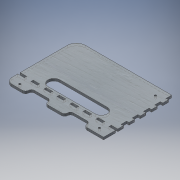
# Autodesk Inventor part: LatoPy
Saved by Autodesk Inventor 2018.3 (Build 223284000, 284)
## iProperties
Created: 2019-03-05
Part Number: LatoPy
Material: Generico
Document SubType Name: Modeling
Designer: AlfyPc
Density: 1 g/cm^3
Appearance: Legno - Verniciato - Bianco
Author: AlfyPc
Autodesk Inventor part; units mm, degrees
ref_plane "YZ Plane" through (0, 0, 0) normal (1, 0, 0) x (0, 1, 0)
ref_plane "XZ Plane" through (0, 0, 0) normal (0, 1, 0) x (-1, 0, 0)
ref_plane "XY Plane" through (0, 0, 0) normal (0, 0, 1) x (1, 0, 0)
sketch "Schizzo1" plane through (0, 0, 0) normal (0, 0, 1) x (1, 0, 0)
  line L0 (4, 17) -> (0, 17) construction
  line L1 (0, 17) -> (0, 95) construction
  line L2 (0, 95) -> (4, 95) construction
  line L3 (4, 95) -> (4, 17) construction
  line L4 (4, -4) -> (4, -24) construction
  line L5 (4, -24) -> (0, -24) construction
  line L6 (0, -24) -> (0, -4) construction
  line L7 (0, 0) -> (0, 11) construction
  line L8 (0, 11) -> (4, 11) construction
  line L9 (4, 11) -> (4, 0) construction
  line L10 (-161, -24) -> (-161, 95)
  line L11 (-161, 95) -> (4, 95)
  line L12 (4, 95) -> (4, -24)
  line L13 (-133, -24) -> (-161, -24)
  arc A0 (-133, -24) -> (-128, -19) centre (-133, -19) ccw
  arc A1 (-123, -14) -> (-128, -19) centre (-123, -19) ccw
  line L14 (-100, -14) -> (-123, -14)
  arc A2 (-95, -19) -> (-100, -14) centre (-100, -19) ccw
  arc A3 (-95, -19) -> (-90, -24) centre (-90, -19) ccw
  line L15 (-67, -24) -> (-90, -24)
  arc A4 (-67, -24) -> (-62, -19) centre (-67, -19) ccw
  arc A5 (-57, -14) -> (-62, -19) centre (-57, -19) ccw
  line L16 (-34, -14) -> (-57, -14)
  arc A6 (-29, -19) -> (-34, -14) centre (-34, -19) ccw
  arc A7 (-29, -19) -> (-24, -24) centre (-24, -19) ccw
  line L17 (4, -24) -> (-24, -24)
  line L18 (-117, 13) -> (-37, 13) construction
  line L19 (-117, 3) -> (-37, 3)
  line L20 (-37, 23) -> (-117, 23)
  arc A8 (-117, 23) -> (-117, 3) centre (-117, 13) ccw
  arc A9 (-37, 3) -> (-37, 23) centre (-37, 13) ccw
  line L21 (-161, -4) -> (-150, -4) projected
  line L22 (-150, 0) -> (-150, -4) projected
  line L23 (-139, -4) -> (-128, -4) projected
  line L24 (-128, 0) -> (-128, -4) projected
  line L25 (-139, 0) -> (-128, 0) projected
  line L26 (-139, 0) -> (-139, -4) projected
  line L27 (-117, -4) -> (-106, -4) projected
  line L28 (-106, 0) -> (-106, -4) projected
  line L29 (-117, 0) -> (-106, 0) projected
  line L30 (-117, 0) -> (-117, -4) projected
  line L31 (-95, -4) -> (-84, -4) projected
  line L32 (-84, 0) -> (-84, -4) projected
  line L33 (-95, 0) -> (-84, 0) projected
  line L34 (-95, 0) -> (-95, -4) projected
  line L35 (-73, -4) -> (-62, -4) projected
  line L36 (-62, 0) -> (-62, -4) projected
  line L37 (-73, 0) -> (-62, 0) projected
  line L38 (-73, 0) -> (-73, -4) projected
  line L39 (-51, -4) -> (-40, -4) projected
  line L40 (-40, 0) -> (-40, -4) projected
  line L41 (-51, 0) -> (-40, 0) projected
  line L42 (-51, 0) -> (-51, -4) projected
  line L43 (-29, -4) -> (-18, -4) projected
  line L44 (-18, 0) -> (-18, -4) projected
  line L45 (-29, 0) -> (-18, 0) projected
  line L46 (-29, 0) -> (-29, -4) projected
  line L47 (-7, -4) -> (4, -4) projected
  line L48 (4, 0) -> (4, -4) projected
  line L49 (-7, 0) -> (4, 0) projected
  line L50 (-7, 0) -> (-7, -4) projected
  line L51 (-161, 0) -> (-150, 0) projected
  line L52 (-161, 0) -> (-161, -4) projected
  point P0 (-77, 13)
  dimension "d0" = 80
  constraints: 44 end point, 20 point on circle, 10 centre point, 6 vertical, 4 horizontal, 4 tangent, 2 parallel, 1 midpoint, 10 other
  measures "d0" distance of L18.start L18.end
extrude "Estrusione1" add sketch "Schizzo1" along normal blind 4 contours L10 L21 L22 L51 L11 L12 L49 L50 L47 L17 A7 A6 L16 A5 A4 L15 A3 A2 L14 A1 A0 L13
sketch "Schizzo2" plane through (0, 0, 4) normal (0, 0, 1) x (1, 0, 0)
  line L0 (0, 76) -> (4, 76)
  line L1 (4, 76) -> (4, 66.5)
  line L2 (4, 66.5) -> (0, 66.5)
  line L3 (0, 66.5) -> (0, 76)
  line L4 (4, 85.5) -> (0, 85.5)
  line L5 (0, 85.5) -> (0, 95)
  line L6 (0, 95) -> (4, 95)
  line L7 (4, 95) -> (4, 85.5)
  line L8 (0, 38) -> (4, 38)
  line L9 (4, 38) -> (4, 28.5)
  line L10 (4, 28.5) -> (0, 28.5)
  line L11 (0, 28.5) -> (0, 38)
  line L12 (4, 47.5) -> (0, 47.5)
  line L13 (0, 47.5) -> (0, 57)
  line L14 (0, 57) -> (4, 57)
  line L15 (4, 57) -> (4, 47.5)
  line L16 (4, 9.5) -> (0, 9.5)
  line L17 (0, 9.5) -> (0, 19)
  line L18 (0, 19) -> (4, 19)
  line L19 (4, 19) -> (4, 9.5)
  point P0 (0, 0)
  constraints: 40 end point, 10 horizontal, 10 vertical, 20 other
extrude "Estrusione2" cut sketch "Schizzo2" against normal blind 4
fillet "Raccordo1" radius 15 1 edges at (-161, 95, 2)
fillet "Raccordo2" radius 10 1 edges at (-161, -24, 2)
sketch "Schizzo3" plane through (0, 0, 4) normal (0, 0, 1) x (1, 0, 0)
  line L0 (-146.15, 0) -> (-142.85, 0) projected
  line L1 (-14.15, 0) -> (-10.85, 0) projected
  line L2 (-144.5, 0) -> (-144.5, -17) construction
  circle A0 centre (-144.5, -17) radius 1.65
  line L3 (0, 79.1) -> (0, 82.4) construction
  line L4 (0, -15.65) -> (0, -12.35) construction
  line L5 (0, -14) -> (-13, -14) construction
  line L6 (0, 80.75) -> (-13, 80.75) construction
  circle A1 centre (-13, 80.75) radius 1.65
  circle A2 centre (-13, -14) radius 1.65
  point P0 (0, 0)
  dimension "d8" = 3.3
  dimension "d13" = 13
  dimension "d14" = 13
  dimension "d15" = 3.3
  dimension "d16" = 3.3
  dimension "d17" = 17
  constraints: 6 end point, 3 centre point, 3 coincident, 3 midpoint, 2 horizontal, 1 vertical
  measures "d8" diameter of A0
  measures "d13" distance of L5.start L5.end
  measures "d14" distance of L6.start L6.end
  measures "d15" diameter of A1
  measures "d16" diameter of A2
  measures "d17" distance of L2.start L2.end
extrude "Estrusione3" cut sketch "Schizzo3" against normal blind 4
